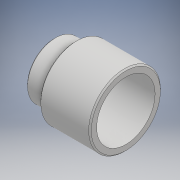
# Autodesk Inventor part: logement roue libre
Saved by Autodesk Inventor 2018.1 (Build 221171000, 171)
## iProperties
Created: 2022-06-29
Part Number: logement roue libre
Material: Generic
Document SubType Name: Modeling
Designer: Bureau
Density: 1 g/cm^3
Appearance: Default
Author: Bureau
Autodesk Inventor part; units mm, degrees
ref_plane "YZ Plane" through (0, 0, 0) normal (1, 0, 0) x (0, 1, 0)
ref_plane "XZ Plane" through (0, 0, 0) normal (0, 1, 0) x (-1, 0, 0)
ref_plane "XY Plane" through (0, 0, 0) normal (0, 0, 1) x (1, 0, 0)
sketch "Sketch1" plane through (0, 0, 0) normal (0, 0, 1) x (1, 0, 0)
  line L0 (0, 0) -> (5, 0)
  line L1 (0, 8.5) -> (0, 10.5)
  line L2 (0, 10.5) -> (8, 10.5)
  line L3 (8, 10.5) -> (8, 13.5)
  line L4 (8, 13.5) -> (27, 13.5)
  line L5 (27, 13.5) -> (27, 11)
  line L6 (27, 11) -> (11, 11)
  line L7 (11, 11) -> (11, 8.5)
  line L8 (11, 8.5) -> (0, 8.5)
  dimension "d0" = 5
  dimension "d1" = 8.5
  dimension "d2" = 2
  dimension "d3" = 8
  dimension "d4" = 3
  dimension "d5" = 19
  dimension "d6" = 2.5
  dimension "d7" = 16
  dimension "d8" = 11
  dimension "d15" = 3
  constraints: 18 end point, 6 perpendicular, 1 horizontal, 1 parallel, 1 vertical
  measures "d0" distance of L0.start L0.end
  measures "d1" distance of L0.start L1.start
  measures "d2" distance of L1.start L1.end
  measures "d3" distance of L1.end L2.end
  measures "d4" distance of L2.end L3.end
  measures "d5" distance of L3.end L4.end
  measures "d6" distance of L4.end L5.end
  measures "d7" distance of L5.end L6.end
  measures "d8" vertical distance of L0.end L5.end
  measures "d15" distance between parallel lines of L7 L3
revolve "Revolution1" add sketch "Sketch1" angle 360 about axis through (0, 0, 0) along (1, 0, 0)
chamfer "Chamfer1" distance 0.5 angle 45 3 edges at (27, -13.5, 0) (8, -13.5, 0) (0, -10.5, 0)
thread "Thread1" size "M16x1" class "6H" standard "ANSI Metric M Profile" full length
body "Solid1"
